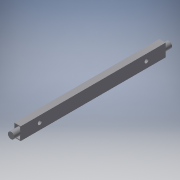
# Autodesk Inventor part: Intake 3 Cross Bar
Saved by Autodesk Inventor 2018 (Build 220112000, 112)
## iProperties
Created: 2018-01-22
Part Number: Intake 3 Cross Bar
Material: Generic
Document SubType Name: Modeling
Designer: Apple
Density: 1 g/cm^3
Appearance: Default
Author: Apple
Autodesk Inventor part; units mm, degrees
ref_plane "YZ Plane" through (0, 0, 0) normal (1, 0, 0) x (0, 1, 0)
ref_plane "XZ Plane" through (0, 0, 0) normal (0, 1, 0) x (-1, 0, 0)
ref_plane "XY Plane" through (0, 0, 0) normal (0, 0, 1) x (1, 0, 0)
sketch "Sketch1" plane through (0, 0, 0) normal (0, 0, 1) x (1, 0, 0)
  line L0 (-26.5191, 402.9946) -> (-1.1191, 402.9946)
  line L1 (-1.1191, 402.9946) -> (-1.1191, 352.1946)
  line L2 (-1.1191, 352.1946) -> (-26.5191, 352.1946)
  line L3 (-26.5191, 352.1946) -> (-26.5191, 402.9946)
  line L4 (-23.3441, 399.8196) -> (-4.2941, 399.8196)
  line L5 (-4.2941, 399.8196) -> (-4.2941, 355.3696)
  line L6 (-4.2941, 355.3696) -> (-23.3441, 355.3696)
  line L7 (-23.3441, 355.3696) -> (-23.3441, 399.8196)
  point P0 (0, 0)
  dimension "d0" = 50.8
  dimension "d1" = 25.4
  dimension "d2" = 3.175
  constraints: 16 end point, 4 parallel, 2 perpendicular, 1 horizontal, 3 other
  measures "d0" distance of L2.end L0.start
  measures "d1" distance of L1.end L2.end
  measures "d2" distance between parallel lines of L3 L7
extrude "Extrusion1" add sketch "Sketch1" along normal blind 577.85
sketch "Sketch2" plane through (0, 0, 0) normal (0, 0, -1) x (-1, 0, 0)
  circle A0 centre (13.8191, 377.5946) radius 12.7
  line L0 (23.3441, 399.8196) -> (23.3441, 355.3696) projected
  line L1 (23.3441, 355.3696) -> (4.2941, 355.3696) projected
  point P0 (0, 0)
  point P1 (23.3441, 377.5946)
  point P2 (13.8191, 355.3696)
  dimension "d6" = 25.4
  constraints: 2 midpoint, 1 centre point, 1 horizontal alignment, 1 vertical alignment
  measures "d6" diameter of A0
extrude "Extrusion2" add sketch "Sketch2" along normal blind 25.4 and the other way blind 603.25
sketch "Sketch4" plane through (-26.5191, 352.1946, 0) normal (-1, 0, 0) x (0, 0, 1)
  circle A0 centre (76.2, 25.4) radius 7.9375
  line L0 (0, 25.4) -> (0, 50.8) projected
  circle A1 centre (501.65, 25.4) radius 7.9375
  point P0 (0, -352.1946)
  dimension "d17" = 15.875
  dimension "d18" = 76.2
  dimension "d19" = 15.875
  dimension "d20" = 501.65
  constraints: 2 centre point, 1 horizontal alignment
  measures "d17" diameter of A0
  measures "d18" distance from line of A0.centre L0
  measures "d19" diameter of A1
  measures "d20" distance of A1.centre L0.start
extrude "Extrusion4" cut sketch "Sketch4" against normal through all
equation "\"d19\" = d17"
body "Solid1"
